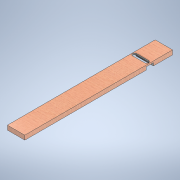
# Autodesk Inventor part: bodyTopPlate
Saved by Autodesk Inventor 2021 (Build 250183000, 183)
## iProperties
Created: 2021-02-01
Part Number: bodyTopPlate
Material: Generic
Document SubType Name: Modeling
Designer: garre
Density: 1 g/cm^3
Appearance: Default
Author: garre
Autodesk Inventor part; units mm, degrees
ref_plane "YZ Plane" through (0, 0, 0) normal (1, 0, 0) x (0, 1, 0)
ref_plane "XZ Plane" through (0, 0, 0) normal (0, 1, 0) x (-1, 0, 0)
ref_plane "XY Plane" through (0, 0, 0) normal (0, 0, 1) x (1, 0, 0)
sketch "Sketch1" plane through (0, 0, 0) normal (0, 1, 0) x (-1, 0, 0)
  line L0 (0, 0) -> (76.2, 0)
  line L1 (76.2, 0) -> (76.2, -647.7)
  line L2 (76.2, -647.7) -> (0, -647.7)
  line L3 (0, -647.7) -> (0, 0)
  dimension "d1" = 76.2
  dimension "d2" = 647.7
  constraints: 8 end point, 2 parallel, 1 horizontal, 1 perpendicular
  measures "d1" distance of L0.start L0.end
  measures "d2" distance of L0.end L1.end
extrude "Extrusion1" add sketch "Sketch1" along normal blind 19.05
sketch "Sketch2" plane through (0, 19.05, 0) normal (0, 1, 0) x (1, 0, 0)
  line L0 (-64.135, 554.99) -> (-12.065, 554.99)
  line L1 (-12.065, 554.99) -> (-12.065, 537.21)
  line L2 (-12.065, 537.21) -> (-64.135, 537.21)
  line L3 (-64.135, 537.21) -> (-64.135, 554.99)
  circle A0 centre (-64.135, 546.1) radius 8.89
  circle A1 centre (-12.065, 546.1) radius 8.89
  line L4 (-73.025, 606.1343) -> (-73.025, 587.8403) construction
  line L5 (-3.175, 554.99) -> (-3.175, 587.8403) construction
  line L6 (0, 647.7) -> (-76.2, 647.7) projected
  line L7 (-38.1, 647.7) -> (-38.1, 0) construction
  line L8 (-76.2, 0) -> (0, 0) projected
  dimension "d5" = 69.85
  dimension "d6" = 34.925
  dimension "d7" = 17.78
  dimension "d8" = 101.6
  constraints: 14 end point, 4 midpoint, 3 vertical, 2 parallel, 2 perpendicular, 1 horizontal, 1 point on line, 6 other
  measures "d5" distance between parallel lines of L4 L5
  measures "d6" distance between parallel lines of L5 L7
  measures "d7" distance of L0.end L1.end
  measures "d8" distance from line of L6 point (-64.135, 546.1)
extrude "Extrusion2" cut sketch "Sketch2" against normal blind 25.4
sketch "Sketch3" plane through (0, 0, 0) normal (0, -1, 0) x (1, 0, 0)
  line L0 (0, 0) -> (0, -647.7) projected
  line L1 (-76.2, -647.7) -> (-76.2, 0) projected
  line L2 (0, -531.3622) -> (-76.2, -531.3622)
  line L3 (-76.2, -531.3622) -> (-76.2, -563.4771)
  line L4 (-76.2, -563.4771) -> (0, -563.4771)
  line L5 (0, -563.4771) -> (0, -531.3622)
  point P0 (0, -563.4771)
  constraints: 8 end point, 2 parallel, 2 point on line, 1 horizontal, 1 perpendicular
extrude "Extrusion3" cut sketch "Sketch3" against normal blind 12.7
equation "\"d1\" = topPlateWidth"
equation "\"d2\" = topPlateLength"
equation "\"d3\" = woodThickness"
equation "\"d6\" = 0.5 * d5"
equation "\"topPlateLength\" = 647.7"
equation "\"woodThickness\" = 19.05"
equation "\"topPlateWidth\" = 76.2"
body "Solid1"
